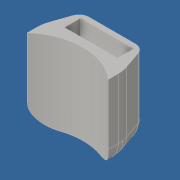
# Autodesk Inventor part: vibramount_v2
Saved by Autodesk Inventor 2016 (Build 200138000, 138)
## iProperties
Created: 2017-05-29
Part Number: vibramount_v2
Material: Generisch
Document SubType Name: Modeling
Designer: 4ndreas
Density: 1 g/cm^3
Appearance: Vorgabe
Author: 4ndreas
Autodesk Inventor part; units mm, degrees
ref_plane "YZ Plane" through (0, 0, 0) normal (1, 0, 0) x (0, 1, 0)
ref_plane "XZ Plane" through (0, 0, 0) normal (0, 1, 0) x (-1, 0, 0)
ref_plane "XY Plane" through (0, 0, 0) normal (0, 0, 1) x (1, 0, 0)
sketch "Skizze1" plane through (0, 0, 0) normal (0, 0, 1) x (1, 0, 0)
  line L0 (-5.25, -1.6) -> (5.25, -1.6)
  line L1 (5.25, -1.6) -> (5.25, 1.6)
  line L2 (5.25, 1.6) -> (-5.25, 1.6)
  line L3 (-5.25, 1.6) -> (-5.25, -1.6)
  line L4 (-5.25, -1.6) -> (5.25, 1.6) construction
  line L5 (5.25, -1.6) -> (-5.25, 1.6) construction
  line L6 (-8, -3.2) -> (8, -3.2)
  line L7 (8, -3.2) -> (6, 2.6)
  line L8 (6, 2.6) -> (-6, 2.6)
  line L9 (-6, 2.6) -> (-8, -3.2)
  line L10 (-8, -3.2) -> (-8, -6.2)
  line L11 (8, -3.2) -> (8, -6.2)
  arc A0 (8, -6.2) -> (-8, -6.2) centre (0, -15.3667) ccw
  line L12 (0, 7.3796) -> (0, -9.7902) construction
  point P0 (0, 0)
  point P1 (0, 0)
  dimension "d0" = 10.5
  dimension "d1" = 3.2
  dimension "d3" = 1
  dimension "d4" = 3
  dimension "d10" = 16
  dimension "d11" = 12
  dimension "d12" = 1.6
  constraints: 26 end point, 4 parallel, 3 midpoint, 3 vertical, 2 horizontal, 2 point on circle, 1 centre point, 1 perpendicular, 1 point on line, 1 tangent, 1 other
  measures "d0" distance between parallel lines of L1 L3
  measures "d1" distance between parallel lines of L0 L2
  measures "d3" distance between parallel lines of L2 L8
  measures "d4" distance of L6.start L10.end
  measures "d10" distance of L6.start L6.end
  measures "d11" distance of L7.end L8.end
  measures "d12" distance between parallel lines of L0 L6
extrude "Extrusion1" add sketch "Skizze1" along normal blind 13
sketch "Skizze2" plane through (0, 0, 0) normal (0, 0, -1) x (-1, 0, 0)
  line L0 (5.25, 1.6) -> (5.25, -1.6) projected
  line L1 (5.25, -1.6) -> (-5.25, -1.6) projected
  line L2 (-5.25, -1.6) -> (-5.25, 1.6) projected
  line L3 (-5.25, 1.6) -> (5.25, 1.6) projected
  line L4 (6, 2.6) -> (8, -3.2) projected
  line L5 (-6, 2.6) -> (6, 2.6) projected
  line L6 (-8, -3.2) -> (-6, 2.6) projected
  arc A0 (8, -6.2) -> (-8, -6.2) centre (0, -15.3667) ccw projected
  line L7 (8, -3.2) -> (8, -6.2) projected
  line L8 (-8, -6.2) -> (-8, -3.2) projected
  point P0 (0, 0)
extrude "Extrusion2" add sketch "Skizze2" along normal blind 3 contours L0 L1 L2 L3 | L4 L7 A0 L8 L6 L5
fillet "Rundung1" radius 2 2 edges at (6, 2.6, 5) (-6, 2.6, 5)
fillet "Rundung1" radius 6 2 edges at (8, -3.2, 5) (-8, -3.2, 5)
fillet "Rundung2" radius 5 2 edges at (-5.25, 0, 0) (5.25, 0, 0)
fillet "Rundung3" radius 4 9 edges at (-7.0685, -0.4988, -3) (-7.9175, -3.2138, -3) (-8, -5.2027, -3) (0, 2.6, -3) (5.7351, 2.2285, -3) (7.0685, -0.4988, -3) (7.9175, -3.2138, -3) (8, -5.2027, -3) (-5.7351, 2.2285, -3)
